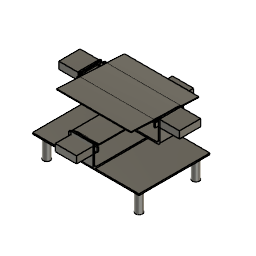
table (Autodesk Fusion 360 design; units mm, degrees)
part number: 2026-04-05-14-13-40-506
Autodesk Fusion 360 part; units mm, degrees
sketch "Sketch1" plane through (0, 0, 0) normal (0, 0, 1) x (1, 0, 0)
  line L0 (0, 0) -> (150, 0)
  line L1 (150, 0) -> (150, 100)
  line L2 (150, 100) -> (0, 100)
  line L3 (0, 100) -> (0, 0)
  circle A0 centre (10, 90) radius 5
  dimension "d1" = 150
  dimension "d2" = 100
  dimension "d3" = 10
  dimension "d4" = 10
  dimension "d5" = 10
  constraint horizontal L0
  constraint vertical L1
  constraint horizontal L2
  constraint vertical L3
  constraint coincident L0.start L3.end
  measures "d1" distance of L0.start L0.end
  measures "d2" distance of L0.start L2.end
  measures "d3" diameter of A0
  measures "d4" distance of L2 A0.centre
  measures "d5" distance of L3 A0.centre
extrude "Extrude1" add sketch "Sketch1" along normal blind 2 contours L0 L1 L2 L3 | A0 makes body 1
sketch "Sketch2" plane through (0, 0, 2) normal (0, 0, 1) x (-1, 0, 0)
  line L0 (0, -100) -> (0, 0)
  line L1 (0, 0) -> (-150, 0)
  line L2 (-150, 0) -> (-150, -100)
  line L3 (-150, -100) -> (0, -100)
  circle A0 centre (-10, -90) radius 5
  circle A1 centre (-140, -90) radius 5
  circle A2 centre (-140, -10) radius 5
  circle A3 centre (-10, -10) radius 5
  dimension "d8" = 10
  dimension "d9" = 10
  dimension "d10" = 10
  dimension "d11" = 10
  dimension "d12" = 10
  dimension "d13" = 10
  dimension "d14" = 10
  dimension "d15" = 10
  dimension "d16" = 10
  dimension "d17" = 10
  dimension "d18" = 10
  dimension "d19" = 10
  measures "d8" diameter of A0
  measures "d9" distance of L3 A0.centre
  measures "d10" distance of L0 A0.centre
  measures "d11" diameter of A1
  measures "d12" distance of L3 A1.centre
  measures "d13" distance of L2 A1.centre
  measures "d14" diameter of A2
  measures "d15" distance of L2 A2.centre
  measures "d16" distance of L1 A2.centre
  measures "d17" diameter of A3
  measures "d18" distance of L0 A3.centre
  measures "d19" distance of L1 A3.centre
extrude "Extrude2" add sketch "Sketch2" along normal blind 30 contours A0 | A1 | A2 | A3 bodies 1
sketch "Sketch3" plane through (0, 0, 0) normal (0, 0, -1) x (1, 0, 0)
  line L0 (0, 0) -> (0, -100)
  line L1 (0, -100) -> (150, -100)
  line L2 (150, -100) -> (150, 0)
  line L3 (150, 0) -> (0, 0)
  line L4 (0, -25) -> (5, -25)
  line L5 (5, -25) -> (5, -75)
  line L6 (5, -75) -> (0, -75)
  line L7 (0, -75) -> (0, -25)
  dimension "d22" = 5
  dimension "d23" = 50
  dimension "d24" = 25
  constraint horizontal L4
  constraint vertical L5
  constraint horizontal L6
  constraint vertical L7
  constraint coincident L0 L4.start
  measures "d22" distance of L4.start L4.end
  measures "d23" distance of L4.start L6.end
  measures "d24" distance of L3 L4
extrude "Extrude3" add sketch "Sketch3" along normal blind 25 contours L0 L4 L5 L6 L7 bodies 1
sketch "Sketch4" plane through (5, 0, 0) normal (1, 0, 0) x (0, 1, 0)
  line L0 (75, 0) -> (25, 0)
  line L1 (25, 0) -> (25, -25)
  line L2 (25, -25) -> (75, -25)
  line L3 (75, -25) -> (75, 0)
  line L4 (65, -17.5) -> (35, -17.5)
  line L5 (35, -17.5) -> (35, -7.5)
  line L6 (35, -7.5) -> (65, -7.5)
  line L7 (65, -7.5) -> (65, -17.5)
  dimension "d27" = 30
  dimension "d28" = 10
  dimension "d29" = 7.5
  dimension "d30" = 10
  constraint horizontal L4
  constraint vertical L5
  constraint horizontal L6
  constraint vertical L7
  measures "d27" distance of L4.start L4.end
  measures "d28" distance of L4.start L6.end
  measures "d29" distance of L2 L4
  measures "d30" distance of L1 L5
extrude "Extrude4" cut sketch "Sketch4" against normal blind 5 contours L4 L5 L6 L7 bodies 1
sketch "Sketch5" plane through (5, 0, 0) normal (1, 0, 0) x (0, 1, 0)
  line L0 (35, -17.5) -> (35, -7.5)
  line L1 (35, -7.5) -> (65, -7.5)
  line L2 (65, -7.5) -> (65, -17.5)
  line L3 (65, -17.5) -> (35, -17.5)
  line L4 (75, 0) -> (25, 0)
  line L5 (25, 0) -> (25, -25)
  line L6 (25, -25) -> (75, -25)
  line L7 (75, -25) -> (75, 0)
  line L8 (65, -17.5) -> (35, -17.5)
  line L9 (35, -17.5) -> (35, -7.5)
  line L10 (35, -7.5) -> (65, -7.5)
  line L11 (65, -7.5) -> (65, -17.5)
  line L12 (35, -15.178) -> (30.036, -15.178)
  line L13 (30.036, -15.178) -> (30.036, -8.9283)
  line L14 (30.036, -8.9283) -> (35, -8.9283)
  line L15 (35, -8.9283) -> (35, -15.178)
  line L16 (65, -15.212) -> (70.0473, -15.212)
  line L17 (70.0473, -15.212) -> (70.0473, -8.9283)
  line L18 (70.0473, -8.9283) -> (65, -8.9283)
  line L19 (65, -8.9283) -> (65, -15.212)
  constraint horizontal L8
  constraint vertical L9
  constraint horizontal L10
  constraint vertical L11
  constraint coincident L0.end L1.start
  constraint coincident L2.end L3.start
  constraint horizontal L12
  constraint vertical L13
  constraint horizontal L14
  constraint vertical L15
  constraint coincident L9 L12.start
  constraint horizontal L16
  constraint vertical L17
  constraint horizontal L18
  constraint vertical L19
  constraint coincident L11 L16.start
extrude "Extrude5" add sketch "Sketch5" along normal blind 2 separate body contours L0 L1 L2 L3 L8 L9 L10 L11 L15 L19 | L0 L9 L12 L13 L14 L15 | L2 L11 L16 L17 L18 L19 makes body 2
sketch "Sketch6" plane through (0, 0, 0) normal (-1, 0, 0) x (0, -1, 0)
  line L0 (-35, -7.5) -> (-35, -17.5)
  line L1 (-35, -17.5) -> (-65, -17.5)
  line L2 (-65, -17.5) -> (-65, -7.5)
  line L3 (-65, -7.5) -> (-35, -7.5)
  line L4 (-100, 0) -> (-75, 0)
  line L5 (-75, 0) -> (-75, -25)
  line L6 (-75, -25) -> (-25, -25)
  line L7 (-25, -25) -> (-25, 0)
  line L8 (-25, 0) -> (0, 0)
  line L9 (0, 0) -> (0, 2)
  line L10 (0, 2) -> (-100, 2)
  line L11 (-100, 2) -> (-100, 0)
  line L12 (-35, -17.5) -> (-65, -17.5)
  line L13 (-65, -17.5) -> (-65, -7.5)
  line L14 (-65, -7.5) -> (-35, -7.5)
  line L15 (-35, -7.5) -> (-35, -17.5)
  constraint horizontal L12
  constraint vertical L13
  constraint horizontal L14
  constraint vertical L15
  constraint coincident L2.end L3.start
  constraint coincident L0.end L1.start
extrude "Extrude6" add sketch "Sketch6" along normal blind 30 separate body contours L0 L1 L2 L3 L12 L13 L14 L15 makes body 3
sketch "Sketch7" plane through (7, 0, 0) normal (1, 0, 0) x (0, 1, 0)
  line L0 (65, -15.212) -> (70.0473, -15.212)
  line L1 (70.0473, -15.212) -> (70.0473, -8.9283)
  line L2 (70.0473, -8.9283) -> (65, -8.9283)
  line L3 (65, -8.9283) -> (65, -7.5)
  line L4 (65, -7.5) -> (35, -7.5)
  line L5 (35, -7.5) -> (35, -8.9283)
  line L6 (35, -8.9283) -> (30.036, -8.9283)
  line L7 (30.036, -8.9283) -> (30.036, -15.178)
  line L8 (30.036, -15.178) -> (35, -15.178)
  line L9 (35, -15.178) -> (35, -17.5)
  line L10 (35, -17.5) -> (65, -17.5)
  line L11 (65, -17.5) -> (65, -15.212)
  circle A0 centre (40.0823, -12.9756) radius 2.9995
extrude "Extrude7" add sketch "Sketch7" along normal blind 2 contours A0 bodies 2
sketch "Sketch8" plane through (9, 0, 0) normal (1, 0, 0) x (0, 1, 0)
  circle A0 centre (40.0823, -12.9756) radius 2.9995
  circle A1 centre (40.0823, -12.9756) radius 1.2467
  line L0 (40.0175, -14.2207) -> (28.6692, -13.6301)
  line L1 (31.1436, -13.2141) -> (39.8757, -11.7462)
  line L2 (40.0201, -14.1708) -> (31.172, -13.7103)
  line L3 (29.1265, -13.6039) -> (39.8839, -11.7954)
  arc A2 (31.1436, -13.2141) -> (31.172, -13.7103) centre (31.185, -13.4606) ccw
  dimension "d40" = 0.25
  constraint concentric A0 A1
  constraint coincident A1 L0.start
  constraint tangent A1 L0
  constraint coincident A1 L1.end
  constraint tangent A1 L1
  constraint coincident L3.start L2
  constraint coincident L0.end L1
  constraint tangent L2 A2
  constraint tangent L1 A2
  measures "d40" radius of A2
extrude "Extrude8" add sketch "Sketch8" along normal blind 2 contours A0 A1 L2 L3 | A0 L2 L3 A2 | A1 bodies 2
sketch "Sketch9" plane through (11, 0, 0) normal (1, 0, 0) x (0, 1, 0)
  arc A0 (39.6712, -14.1526) -> (39.5394, -11.8534) centre (40.0823, -12.9756) ccw
  line L0 (39.5394, -11.8534) -> (31.004, -13.2882)
  arc A1 (31.004, -13.2882) -> (31.172, -13.7103) centre (31.185, -13.4606) ccw
  line L1 (31.172, -13.7103) -> (39.6712, -14.1526)
  line L2 (44.9407, -19.0545) -> (-14.5856, -19.0545)
  line L3 (-14.5856, -19.0545) -> (-14.5856, -6.5594)
  line L4 (-14.5856, -6.5594) -> (44.9407, -6.5594)
  line L5 (44.9407, -6.5594) -> (44.9407, -19.0545)
  constraint horizontal L2
  constraint vertical L3
  constraint horizontal L4
  constraint vertical L5
extrude "Extrude9" add sketch "Sketch9" along normal blind 1 separate body makes body 4
move_body "Move1" bodies 4 to x (1, 0, 0) y (0, 1, 0) z (0, 0, 1) at (-2, 0, 0)
copy_body "CopyPasteBodies1" bodies 4 makes body 5
sketch "Sketch10" plane through (10, 0, 0) normal (1, 0, 0) x (0, 1, 0)
  line L0 (39.6712, -14.1526) -> (31.172, -13.7103)
  arc A0 (31.004, -13.2882) -> (31.172, -13.7103) centre (31.185, -13.4606) ccw
  line L1 (31.004, -13.2882) -> (39.5394, -11.8534)
  arc A1 (39.6712, -14.1526) -> (39.5394, -11.8534) centre (40.0823, -12.9756) ccw
  line L2 (44.9407, -6.5594) -> (-14.5856, -6.5594)
  line L3 (-14.5856, -6.5594) -> (-14.5856, -19.0545)
  line L4 (-14.5856, -19.0545) -> (44.9407, -19.0545)
  line L5 (44.9407, -19.0545) -> (44.9407, -6.5594)
  line L6 (-14.5856, -19.0545) -> (-12.509, -19.0545)
  line L7 (-12.509, -19.0545) -> (-12.509, -6.5594)
  line L8 (-12.509, -6.5594) -> (-14.5856, -6.5594)
  line L9 (-14.5856, -6.5594) -> (-14.5856, -19.0545)
  constraint horizontal L6
  constraint vertical L7
  constraint horizontal L8
  constraint vertical L9
  constraint coincident L2 L7.end
  constraint coincident L3.end L4.start
extrude "Extrude10" add sketch "Sketch10" along normal blind 65 contours L2 L3 L4 L6 L7 L8 L9 bodies 4 5
copy_body "CopyPasteBodies2" bodies 3 makes body 6
move_body "Move2" bodies 6 to x (0, 1, 0) y (-1, 0, 0) z (0, 0, 1) at (105, -13, 0)
copy_body "CopyPasteBodies3" bodies 2 makes body 7
move_body "Move3" bodies 7 to x (0, 1, 0) y (-1, 0, 0) z (0, 0, 1) at (105.036, -14.964, 0)
move_body "Move4" bodies 7 to x (1, 0, 0) y (0, 1, 0) z (0, 0, 1) at (0, -3, 0)
sketch "Sketch11" plane through (0, -6.964, 0) normal (0, 1, 0) x (-1, 0, 0)
  arc A0 (-65.3648, -14.1526) -> (-65.4967, -11.8534) centre (-64.9537, -12.9756) ccw
  line L0 (-65.4967, -11.8534) -> (-74.032, -13.2882)
  arc A1 (-74.032, -13.2882) -> (-73.864, -13.7103) centre (-73.851, -13.4606) ccw
  line L1 (-73.864, -13.7103) -> (-65.3648, -14.1526)
  line L2 (-55.009, -16.0098) -> (-80.0535, -16.0098)
  line L3 (-80.0535, -16.0098) -> (-80.0535, -9.9384)
  line L4 (-80.0535, -9.9384) -> (-55.009, -9.9384)
  line L5 (-55.009, -9.9384) -> (-55.009, -16.0098)
  constraint horizontal L2
  constraint vertical L3
  constraint horizontal L4
  constraint vertical L5
extrude "Extrude11" add sketch "Sketch11" along normal blind 1 separate body makes body 8
move_body "Move5" bodies 8 to x (1, 0, 0) y (0, 1, 0) z (0, 0, 1) at (0, -2, 0)
sketch "Sketch12" plane through (0, 0, -16.0098) normal (0, 0, -1) x (1, 0, 0)
  line L0 (80.0535, 8.964) -> (55.009, 8.964)
  line L1 (55.009, 8.964) -> (55.009, 7.964)
  line L2 (55.009, 7.964) -> (80.0535, 7.964)
  line L3 (80.0535, 7.964) -> (80.0535, 8.964)
  line L4 (44.8605, 9.886) -> (130.8207, 9.886)
  line L5 (130.8207, 9.886) -> (130.8207, -50.6508)
  line L6 (130.8207, -50.6508) -> (44.8605, -50.6508)
  line L7 (44.8605, -50.6508) -> (44.8605, 9.886)
  constraint horizontal L4
  constraint vertical L5
  constraint horizontal L6
  constraint vertical L7
extrude "Extrude12" add sketch "Sketch12" along normal blind 5 contours L0 L1 L2 L3 | L4 L5 L6 L7 bodies 8
sketch "Sketch13" plane through (0, 0, 0) normal (0, 0, 1) x (1, 0, 0)
  line L0 (30.0777, 24.6506) -> (145.2374, 24.6506)
  line L1 (145.2374, 24.6506) -> (145.2374, 55.7817)
  line L2 (145.2374, 55.7817) -> (30.0777, 55.7817)
  line L3 (30.0777, 55.7817) -> (30.0777, 24.6506)
  constraint horizontal L0
  constraint vertical L1
  constraint horizontal L2
  constraint vertical L3
extrude "Extrude13" add sketch "Sketch13" against normal blind 2 separate body makes body 9
sketch "Sketch14" plane through (0, 0, -2) normal (0, 0, -1) x (1, 0, 0)
  line L0 (30.0777, -24.6506) -> (30.0777, -55.7817)
  line L1 (30.0777, -55.7817) -> (145.2374, -55.7817)
  line L2 (145.2374, -55.7817) -> (145.2374, -24.6506)
  line L3 (145.2374, -24.6506) -> (30.0777, -24.6506)
  line L4 (30.0777, -55.7817) -> (32.0777, -55.7817)
  line L5 (32.0777, -55.7817) -> (32.0777, -24.6506)
  line L6 (32.0777, -24.6506) -> (30.0777, -24.6506)
  line L7 (30.0777, -24.6506) -> (30.0777, -55.7817)
  line L8 (145.2374, -55.7817) -> (143.2374, -55.7817)
  line L9 (143.2374, -55.7817) -> (143.2374, -24.6506)
  line L10 (143.2374, -24.6506) -> (145.2374, -24.6506)
  line L11 (145.2374, -24.6506) -> (145.2374, -55.7817)
  dimension "d53" = 2
  dimension "d54" = 2
  constraint horizontal L4
  constraint vertical L5
  constraint horizontal L6
  constraint vertical L7
  constraint coincident L3 L5.end
  constraint coincident L0.end L1.start
  constraint horizontal L8
  constraint vertical L9
  constraint horizontal L10
  constraint vertical L11
  constraint coincident L3 L9.end
  constraint coincident L1.end L2.start
  measures "d53" distance of L0.end L4.end
  measures "d54" distance of L1.end L8.end
extrude "Extrude14" add sketch "Sketch14" along normal blind 30 contours L0 L1 L3 L4 L5 L6 L7 | L1 L2 L3 L8 L9 L10 L11 bodies 9
fillet "Fillet1" radius 2.5 1 edges at (145.2374, 40.2161, 0) on bodies 9
fillet "Fillet2" radius 2.5 1 edges at (30.0777, 40.2161, 0) on bodies 9
fillet "Fillet3" radius 2.5 1 edges at (32.0777, 40.2161, -2) on bodies 9
fillet "Fillet4" radius 2.5 1 edges at (143.2374, 40.2161, -2) on bodies 9
copy_body "CopyPasteBodies4" bodies 2 makes body 10
move_body "Move6" bodies 10 to x (-1, 0, 0) y (0, -1, 0) z (0, 0, 1) at (135, 60.0721, 0)
move_body "Move7" bodies 10 to x (1, 0, 0) y (0, 1, 0) z (0, 0, 1) at (0, 10, -13)
move_body "Move8" bodies 10 to x (1, 0, 0) y (0, 1, 0) z (0, 0, 1) at (13, 0, 0)
move_body "Move9" bodies 10 to x (1, 0, 0) y (0, 1, 0) z (0, 0, 1) at (0, 20, 0)
copy_body "CopyPasteBodies5" bodies 10 makes body 11
move_body "Move10" bodies 11 to x (-1, 0, 0) y (0, -1, 0) z (0, 0, 1) at (164, 40.0495, 0)
move_body "Move11" bodies 11 to x (1, 0, 0) y (0, 1, 0) z (0, 0, 1) at (11, 40, 0)
sketch "Sketch15" plane through (0, -1.3292, -25.5404) normal (0, -0.051973, -0.998648) x (1, 0, 0)
  line L0 (36, -28.6187) -> (36, -31.0198)
  line L1 (36, -31.0198) -> (38, -31.0198)
  line L2 (38, -31.0198) -> (38, -22.5091)
  line L3 (38, -22.5091) -> (36, -22.5091)
  line L4 (36, -22.5091) -> (36, -28.6187)
  line L5 (36, -22.5091) -> (139.2378, -22.5091)
  line L6 (139.2378, -22.5091) -> (139.2378, -60.3411)
  line L7 (139.2378, -60.3411) -> (36, -60.3411)
  line L8 (36, -60.3411) -> (36, -22.5091)
  constraint horizontal L5
  constraint vertical L6
  constraint horizontal L7
  constraint vertical L8
  constraint coincident L3.end L4.start
extrude "Extrude15" add sketch "Sketch15" 1 faces at (37.3333, 26.0163, -26.9636) along normal blind 1 contours L1 L2 L5 L6 L7 L8 on bodies 11 bodies 10 11
sketch "Sketch16" plane through (0, 0, -25) normal (0, 0, -1) x (1, 0, 0)
  line L0 (0, -75) -> (5, -75)
  line L1 (5, -75) -> (5, -25)
  line L2 (5, -25) -> (0, -25)
  line L3 (0, -25) -> (0, -75)
  line L4 (0, -25) -> (5, -25)
  line L5 (5, -25) -> (5, -75)
  line L6 (5, -75) -> (0, -75)
  line L7 (0, -75) -> (0, -25)
  constraint horizontal L4
  constraint vertical L5
  constraint horizontal L6
  constraint vertical L7
  constraint coincident L0.end L1.start
  constraint coincident L2.end L3.start
extrude "Extrude16" cut sketch "Sketch16" against normal blind 30 bodies 1
sketch "Sketch17" plane through (0, 0, 2) normal (0, 0, 1) x (-1, 0, 0)
  line L0 (-5, -25) -> (0, -25)
  line L1 (0, -25) -> (0, 0)
  line L2 (0, 0) -> (-150, 0)
  line L3 (-150, 0) -> (-150, -100)
  line L4 (-150, -100) -> (0, -100)
  line L5 (0, -100) -> (0, -75)
  line L6 (0, -75) -> (-5, -75)
  line L7 (-5, -75) -> (-5, -25)
  circle A0 centre (-10, -10) radius 5
  circle A1 centre (-10, -90) radius 5
  circle A2 centre (-140, -10) radius 5
  circle A3 centre (-140, -90) radius 5
  line L8 (0, -75) -> (-5, -75)
  line L9 (-5, -75) -> (-5, -25)
  line L10 (-5, -25) -> (0, -25)
  line L11 (0, -25) -> (0, -75)
  constraint horizontal L8
  constraint vertical L9
  constraint horizontal L10
  constraint vertical L11
  constraint coincident L0.start L7.end
  constraint coincident L5.end L6.start
extrude "Extrude17" add sketch "Sketch17" against normal blind 2 contours L0 L6 L7 L8 L9 L10 L11 bodies 1
move_body "Move12" bodies 9 10 to x (1, 0, 0) y (0, 1, 0) z (0, 0, 1) at (-10, 0, -30)
copy_body "CopyPasteBodies6" bodies 9 makes body 12
move_body "Move13" bodies 12 to x (0, 1, 0) y (-1, 0, 0) z (0, 0, 1) at (128.0835, -32.0634, 30)
copy_body "CopyPasteBodies7" bodies 10 makes body 13
copy_body "CopyPasteBodies8" bodies 10 makes body 14
move_body "Move14" bodies 14 to x (0, -1, 0) y (1, 0, 0) z (0, 0, 1) at (46.9866, 123.0134, 30)
move_body "Move15" bodies 12 14 to x (1, 0, 0) y (0, 1, 0) z (0, 0, 1) at (-15, 0, 0)
move_body "Move16" bodies 3 to x (1, 0, 0) y (0, 1, 0) z (0, 0, 1) at (87, -75, -10)
copy_body "CopyPasteBodies9" bodies 3 makes body 15
move_body "Move17" bodies 15 to x (1, 0, 0) y (0, 1, 0) z (0, 0, 1) at (0, 135, 0)
copy_body "CopyPasteBodies10" bodies 3 makes body 16
move_body "Move18" bodies 16 to x (1, 0, 0) y (0, 1, 0) z (0, 0, 1) at (-58, 63, -13)
move_body "Move19" bodies 16 to x (1, 0, 0) y (0, 1, 0) z (0, 0, 1) at (-10, 0, -20)
move_body "Move20" bodies 16 to x (1, 0, 0) y (0, 1, 0) z (0, 0, 1) at (3, 0, 0)
move_body "Move21" bodies 16 to x (1, 0, 0) y (0, 1, 0) z (0, 0, 1) at (0, 2, 0)
copy_body "CopyPasteBodies11" bodies 16 makes body 17
move_body "Move22" bodies 17 to x (1, 0, 0) y (0, 1, 0) z (0, 0, 1) at (140, 0, 0)
sketch "Sketch18" plane through (0, -2.9383, -56.458) normal (0, -0.051973, -0.998648) x (1, 0, 0)
  line L0 (26, -61.9003) -> (129.2378, -61.9003)
  line L1 (129.2378, -61.9003) -> (129.2378, -24.0683)
  line L2 (129.2378, -24.0683) -> (26, -24.0683)
  line L3 (26, -24.0683) -> (26, -30.886)
  line L4 (26, -30.886) -> (26, -34.9708)
  line L5 (26, -34.9708) -> (26, -61.9003)
  line L6 (26, 0.4807) -> (131.0006, 0.4807)
  line L7 (131.0006, 0.4807) -> (131.0006, -95.4261)
  line L8 (131.0006, -95.4261) -> (26, -95.4261)
  line L9 (26, -95.4261) -> (26, 0.4807)
  constraint horizontal L6
  constraint vertical L7
  constraint horizontal L8
  constraint vertical L9
extrude "Extrude18" add sketch "Sketch18" along normal blind 1 bodies 10 16 17 13
move_body "Move23" bodies 1 2 3 4 6 7 8 9 10 12 14 15 16 17 to x (1, 0, 0) y (0, -1, 0) z (0, 0, -1) at (0, 0, 0)
hidden bodies 2 4 6 7 8
